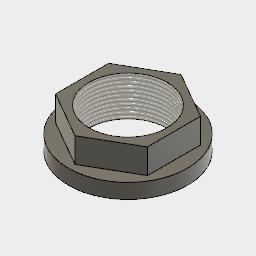
bottoncover v0 (Autodesk Fusion 360 design; units mm, degrees)
Autodesk Fusion 360 part; units mm, degrees
note: some values were not read from the file. Set by a fixed rule: which face or edge a step refers to.
sketch "スケッチ1" plane through (0, 0, 0) normal (0, 1, 0) x (1, 0, 0)
  line L0 (-18.5, -10.681) -> (0, -21.362)
  line L1 (0, -21.362) -> (18.5, -10.681)
  line L2 (18.5, -10.681) -> (18.5, 10.681)
  line L3 (18.5, 10.681) -> (0, 21.362)
  line L4 (0, 21.362) -> (-18.5, 10.681)
  line L5 (-18.5, 10.681) -> (-18.5, -10.681)
  line L6 (0, -20, 20) -> (0, -2.5, 20)
  line L7 (1.75, 0) -> (22.5, 0)
  dimension "d7" = 37
  measures "d7" distance of L2 L5
extrude "押し出し1" add sketch "スケッチ1" along normal blind 10
sketch "スケッチ3" plane through (0, 0, 0) normal (0, 1, 0) x (1, 0, 0)
  circle A0 centre (0, 0) radius 24
  dimension "d8" = 48
  measures "d8" diameter of A0
extrude "押し出し3" add sketch "スケッチ3" against normal blind 6
sketch "スケッチ4" plane through (0, 0, 0) normal (0, 1, 0) x (-1, 0, 0)
  circle A0 centre (0, 0) radius 24
  line L0 (18.5, -10.681) -> (0, -21.362)
  line L1 (0, -21.362) -> (-18.5, -10.681)
  line L2 (-18.5, -10.681) -> (-18.5, 10.681)
  line L3 (-18.5, 10.681) -> (0, 21.362)
  line L4 (0, 21.362) -> (18.5, 10.681)
  line L5 (18.5, 10.681) -> (18.5, -10.681)
  circle A1 centre (0, 0) radius 16.5
  dimension "d11" = 33
  measures "d11" diameter of A1
extrude "押し出し4" cut sketch "スケッチ4" along normal mid plane 32 contours A1
thread "ねじ2" "ISO Metric profile 33.0 M33x1.5 6H" major diameter 33.2083 minor diameter 31.5262 pitch 1.5 angle 60 resizes the face on face at (-16.418, 6.6667, 1.6429) on face at (-16.418, -2, -1.6429)
